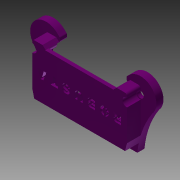
# Autodesk Inventor part: bawahbelakangbaru
Saved by Autodesk Inventor 2015 (Build 190159000, 159)
## iProperties
Created: 2015-01-14
Part Number: bawahbelakangbaru
Material: Generic
Document SubType Name: Modeling
Designer: Rafi Kurnia Putra
Density: 1 g/cm^3
Appearance: Smooth - Purple
Author: Rafi Kurnia Putra
Autodesk Inventor part; units mm, degrees
ref_plane "XY Plane" through (0, 0, 0) normal (0, 0, 1) x (1, 0, 0)
ref_plane "Work Plane2" through (0, -8.5, 0) normal (0, 1, 0) x (-1, 0, 0)
sketch "Sketch12" plane through (0, -8.5, 0) normal (0, 1, 0) x (-1, 0, 0)
  arc A0 (-42.164541, 21.859238) -> (-43.399977, 26.523474) centre (-134.113763, 0) ccw
  line L0 (0.000001, 18.359238) -> (-41.402253, 18.359238)
  arc A1 (-44.972913, 18.359238) -> (-46.899977, 26.017459) centre (-134.113763, 0) ccw
  line L1 (-43.399977, 53.851002) -> (-43.399977, 26.523474)
  line L2 (-46.899977, 36.417593) -> (-46.899977, 56.643984)
  arc A2 (-43.399977, 53.851002) -> (-40.169234, 65.136621) centre (-46.649977, 60.886625) ccw
  line L3 (-40.169234, 65.136621) -> (-34.950271, 65.136621)
  line L4 (-46.764402, 66.336532) -> (-46.764402, 65.135084)
  line L5 (-44.766541, 68.336531) -> (-36.708427, 68.345149)
  arc A3 (-44.766541, 68.336531) -> (-46.764402, 66.336532) centre (-44.764402, 66.336532) ccw
  arc A4 (-36.708427, 68.345149) -> (-33.606775, 65.655062) centre (0.000005, 107.536576) ccw
  arc A5 (-34.950271, 65.136621) -> (-33.606775, 65.655062) centre (-34.950271, 67.136621) ccw
  line L6 (0, 0) -> (0, 3.949172) construction
  line L7 (-0.000001, 18.359238) -> (41.402253, 18.359238)
  arc A6 (46.899977, 26.017459) -> (44.972913, 18.359238) centre (134.113763, 0) ccw
  line L8 (43.399977, 53.851002) -> (43.399977, 26.523474)
  line L9 (46.899977, 36.417593) -> (46.899977, 56.643984)
  arc A7 (40.169234, 65.136621) -> (43.399977, 53.851002) centre (46.649977, 60.886625) ccw
  arc A8 (46.764402, 65.135084) -> (46.899977, 56.643984) centre (46.649977, 60.886624) ccw
  line L10 (40.169234, 65.136621) -> (34.950271, 65.136621)
  line L11 (46.764402, 66.336532) -> (46.764402, 65.135084)
  line L12 (44.766541, 68.336531) -> (36.708427, 68.345149)
  arc A9 (46.764402, 66.336532) -> (44.766541, 68.336531) centre (44.764402, 66.336532) ccw
  arc A10 (33.606775, 65.655062) -> (36.708427, 68.345149) centre (-0.000005, 107.536576) ccw
  arc A11 (33.606775, 65.655062) -> (34.950271, 65.136621) centre (34.950271, 67.136621) ccw
  line L13 (-46.899977, 36.417593) -> (-46.899977, 26.017459)
  line L14 (-44.972913, 18.359238) -> (-41.402253, 18.359238)
  line L15 (41.402253, 18.359238) -> (44.972913, 18.359238)
  line L16 (0.000001, 21.859238) -> (-41.402253, 21.859238)
  line L17 (-0.000001, 21.859238) -> (41.402253, 21.859238)
  line L18 (-41.402253, 21.859238) -> (-42.164541, 21.859238)
  line L19 (41.402253, 21.859238) -> (42.164541, 21.859238)
  arc A12 (43.399977, 26.523474) -> (42.164541, 21.859238) centre (134.113763, 0) ccw
  line L20 (46.899977, 36.417593) -> (46.899977, 26.017459)
  arc A13 (-46.899977, 56.643984) -> (-46.764402, 65.135084) centre (-46.649977, 60.886624) ccw
  line L21 (-44.972913, 18.359238) -> (44.972913, 18.359238)
  line L22 (-42.164541, 21.859238) -> (42.164541, 21.859238)
  arc A14 (-44.972913, 18.359238) -> (-46.899977, 26.017459) centre (-134.113763, 0) ccw
  line L23 (-46.899977, 26.017459) -> (-46.899977, 56.643984)
  arc A15 (-46.899977, 56.643984) -> (-46.764402, 65.135084) centre (-46.649977, 60.886624) ccw
  line L24 (-46.764402, 65.135084) -> (-46.764402, 66.336532)
  arc A16 (-44.766541, 68.336531) -> (-46.764402, 66.336532) centre (-44.764402, 66.336532) ccw
  line L25 (-44.766541, 68.336531) -> (-36.708427, 68.345149)
  arc A17 (-36.708427, 68.345149) -> (-33.606775, 65.655062) centre (0.000005, 107.536576) ccw
  arc A18 (-34.950271, 65.136621) -> (-33.606775, 65.655062) centre (-34.950271, 67.136621) ccw
  line L26 (-34.950271, 65.136621) -> (-40.169234, 65.136621)
  arc A19 (-43.399977, 53.851002) -> (-40.169234, 65.136621) centre (-46.649977, 60.886625) ccw
  line L27 (-43.399977, 53.851002) -> (-43.399977, 26.523474)
  arc A20 (-42.164541, 21.859238) -> (-43.399977, 26.523474) centre (-134.113763, 0) ccw
  line L28 (-42.164541, 21.859238) -> (42.164541, 21.859238)
  arc A21 (43.399977, 26.523465) -> (42.164541, 21.859238) centre (134.110216, 0.000886) ccw
  line L29 (43.399977, 26.523465) -> (43.399977, 53.851002)
  arc A22 (40.169234, 65.136621) -> (43.399977, 53.851002) centre (46.649977, 60.886625) ccw
  line L30 (40.169234, 65.136621) -> (34.950271, 65.136621)
  arc A23 (33.606775, 65.655062) -> (34.950271, 65.136621) centre (34.950271, 67.136621) ccw
  arc A24 (33.606775, 65.655062) -> (36.708427, 68.345149) centre (-0.000005, 107.536576) ccw
  line L31 (36.708427, 68.345149) -> (44.766541, 68.336531)
  arc A25 (46.764402, 66.336532) -> (44.766541, 68.336531) centre (44.764402, 66.336532) ccw
  line L32 (46.764402, 66.336532) -> (46.764402, 65.135084)
  arc A26 (46.764402, 65.135084) -> (46.899977, 56.643984) centre (46.649977, 60.886624) ccw
  line L33 (46.899977, 56.643984) -> (46.899977, 26.017459)
  arc A27 (46.899977, 26.017459) -> (44.972913, 18.359238) centre (134.113763, 0) ccw
  line L34 (44.972913, 18.359238) -> (-44.972913, 18.359238)
  point P0 (0.000002, 53.838562)
  point P1 (-43.59264, 9.438181)
  point P2 (-46.649977, 60.886624)
  point P3 (37.970237, 69.566356)
  point P4 (-0.000002, 53.838562)
  point P5 (43.59264, 9.438181)
  point P6 (43.399975, 60.886623)
  constraints: 72 end point, 57 point on circle, 28 centre point, 22 symmetric about line, 9 tangent, 8 horizontal, 8 vertical, 4 collinear, 3 concentric, 3 parallel, 2 coincident, 1 point on line, 5 other
ref_plane "Work Plane3" through (0, -5, 0) normal (0, 1, 0) x (-1, 0, 0)
sketch "Sketch13" plane through (0, -5, 0) normal (0, 1, 0) x (-1, 0, 0)
  arc A0 (-37.970238, 69.566357) -> (-55.329713, 52.206889) centre (-46.649975, 60.886623) ccw
  arc A1 (-37.970238, 69.566357) -> (-55.329713, 52.206889) centre (-46.649975, 60.886623) ccw
  circle A2 centre (-46.649975, 60.886623) radius 3.25
  arc A3 (-40.074374, 9.438181) -> (-55.329713, 52.206889) centre (-134.113762, -0.000001) ccw
  line L0 (0.000004, 9.438181) -> (-40.074374, 9.438181)
  line L1 (0.000002, 18.359238) -> (-41.402252, 18.359238)
  arc A4 (-35.495359, 72.041226) -> (-33.611129, 70.252097) centre (0.000004, 107.536577) ccw
  arc A5 (-35.495359, 72.041226) -> (-58.067687, 50.001472) centre (-46.649975, 60.886623) ccw
  arc A6 (-43.59264, 9.438181) -> (-58.067687, 50.001472) centre (-134.113762, -0.000001) ccw
  line L2 (-43.59264, 9.438181) -> (-40.074374, 9.438181)
  line L3 (-43.399975, 53.851) -> (-43.399975, 26.523472)
  line L4 (-46.899975, 36.417593) -> (-46.899975, 56.643983)
  arc A7 (-43.399975, 53.851) -> (-40.169234, 65.136621) centre (-46.649975, 60.886623) ccw
  circle A8 centre (-46.649977, 60.886624) radius 4.25
  line L5 (-40.169234, 65.136621) -> (-34.950271, 65.136621)
  line L6 (-46.764402, 66.336532) -> (-46.764402, 65.135084)
  line L7 (-44.766541, 68.336531) -> (-36.708427, 68.345149)
  arc A9 (-44.766541, 68.336531) -> (-46.764402, 66.336532) centre (-44.764402, 66.336532) ccw
  line L8 (-32.950271, 67.136621) -> (-32.950271, 68.766601)
  arc A10 (-37.970238, 69.566357) -> (-33.606774, 65.655062) centre (0.000004, 107.536577) ccw
  arc A11 (-32.950271, 68.766601) -> (-33.611129, 70.252097) centre (-34.950271, 68.766601) ccw
  arc A12 (-34.950271, 65.136621) -> (-32.950271, 67.136621) centre (-34.950271, 67.136621) ccw
  line L9 (0, 0) -> (0, 3.949172) construction
  arc A13 (32.950271, 67.136621) -> (34.950271, 65.136621) centre (34.950271, 67.136621) ccw
  arc A14 (33.611129, 70.252097) -> (35.495359, 72.041226) centre (-0.000004, 107.536577) ccw
  line L10 (32.950271, 67.136621) -> (32.950271, 68.766601)
  arc A15 (33.611129, 70.252097) -> (32.950271, 68.766601) centre (34.950271, 68.766601) ccw
  arc A16 (33.606774, 65.655062) -> (37.970238, 69.566357) centre (-0.000004, 107.536577) ccw
  arc A17 (55.329713, 52.206889) -> (37.970238, 69.566357) centre (46.649975, 60.886623) ccw
  arc A18 (55.329713, 52.206889) -> (37.970238, 69.566357) centre (46.649975, 60.886623) ccw
  line L11 (40.169234, 65.136621) -> (34.950271, 65.136621)
  line L12 (44.766541, 68.336531) -> (36.708427, 68.345149)
  arc A19 (46.764402, 66.336532) -> (44.766541, 68.336531) centre (44.764402, 66.336532) ccw
  line L13 (46.764402, 66.336532) -> (46.764402, 65.135084)
  arc A20 (40.169234, 65.136621) -> (43.399975, 53.851) centre (46.649975, 60.886623) ccw
  circle A21 centre (46.649975, 60.886623) radius 3.25
  circle A22 centre (46.649977, 60.886624) radius 4.25
  arc A23 (58.067687, 50.001472) -> (35.495359, 72.041226) centre (46.649975, 60.886623) ccw
  arc A24 (55.329713, 52.206889) -> (40.074374, 9.438181) centre (134.113762, -0.000001) ccw
  line L14 (-0.000004, 9.438181) -> (40.074374, 9.438181)
  line L15 (-0.000002, 18.359238) -> (41.402252, 18.359238)
  line L16 (46.899975, 36.417593) -> (46.899975, 56.643983)
  line L17 (43.399975, 53.851) -> (43.399975, 26.523472)
  line L18 (43.59264, 9.438181) -> (40.074374, 9.438181)
  arc A25 (58.067687, 50.001472) -> (43.59264, 9.438181) centre (134.113762, -0.000001) ccw
  point P0 (0.000002, 53.838562)
  point P1 (-32.950271, 69.666799)
  point P2 (-43.399975, 60.886623)
  point P3 (32.950271, 69.666799)
  point P4 (43.399975, 60.886623)
  point P5 (-0.000002, 53.838562)
  constraints: 54 point on circle, 40 symmetric about line, 38 end point, 22 centre point, 12 coincident, 6 tangent, 5 vertical, 2 horizontal alignment, 2 point on line, 1 concentric, 1 horizontal, 21 other
extrude "Extrusion9" add sketch "Sketch13" along normal mid plane 7 contours A0 A3 L2 A6 A5 A4 A11 L8 A12 A10 | A24 A17 A16 A13 L10 A15 A14 A23 A25 L18
sketch "Sketch14" plane through (0, -8.5, 0) normal (0, -1, 0) x (1, 0, 0)
  line L0 (40.074374, 9.438181) -> (-40.074374, 9.438181)
  line L1 (-0.000002, 18.359238) -> (41.402252, 18.359238)
  line L2 (0.000002, 18.359238) -> (-41.402252, 18.359238)
  line L3 (-41.402252, 18.359238) -> (41.402252, 18.359238)
  arc A0 (55.329713, 52.206889) -> (40.074374, 9.438181) centre (134.113762, -0.000001) ccw
  line L4 (46.899975, 36.417593) -> (46.899975, 56.643983)
  line L5 (43.399975, 53.851) -> (43.399975, 26.523472)
  arc A1 (55.329713, 52.206889) -> (37.970238, 69.566357) centre (46.649975, 60.886623) ccw
  line L6 (44.766541, 68.336531) -> (36.708427, 68.345149)
  arc A2 (46.764402, 66.336532) -> (44.766541, 68.336531) centre (44.764402, 66.336532) ccw
  line L7 (46.764402, 66.336532) -> (46.764402, 65.135084)
  circle A3 centre (46.649975, 60.886623) radius 3.25
  arc A4 (33.606774, 65.655062) -> (37.970238, 69.566357) centre (-0.000004, 107.536577) ccw
  arc A5 (40.169234, 65.136621) -> (43.399975, 53.851) centre (46.649975, 60.886623) ccw
  line L8 (40.169234, 65.136621) -> (34.950271, 65.136621)
  arc A6 (33.606774, 65.655062) -> (34.950271, 65.136621) centre (34.950271, 67.136621) ccw
  arc A7 (55.329713, 52.206889) -> (40.074374, 9.438181) centre (134.113762, -0.000001) ccw
  arc A8 (-40.074374, 9.438181) -> (-55.329712, 52.206889) centre (-134.113762, -0.000001) ccw
  line L9 (-46.899975, 36.417593) -> (-46.899975, 56.643983)
  line L10 (-43.399975, 53.851) -> (-43.399975, 26.523472)
  arc A9 (-37.970238, 69.566357) -> (-55.329712, 52.206889) centre (-46.649975, 60.886623) ccw
  line L11 (-44.766541, 68.336531) -> (-36.708427, 68.345149)
  arc A10 (-44.766541, 68.336531) -> (-46.764401, 66.336532) centre (-44.764401, 66.336532) ccw
  line L12 (-46.764401, 66.336532) -> (-46.764401, 65.135084)
  circle A11 centre (-46.649975, 60.886623) radius 3.25
  arc A12 (-37.970238, 69.566357) -> (-33.606774, 65.655062) centre (0.000004, 107.536577) ccw
  arc A13 (-43.399975, 53.851) -> (-40.169234, 65.136621) centre (-46.649975, 60.886623) ccw
  line L13 (-40.169234, 65.136621) -> (-34.950271, 65.136621)
  arc A14 (-34.950271, 65.136621) -> (-33.606774, 65.655062) centre (-34.950271, 67.136621) ccw
  arc A15 (-40.074374, 9.438181) -> (-55.329712, 52.206889) centre (-134.113762, -0.000001) ccw
  arc A16 (46.764402, 65.135084) -> (46.899975, 56.643983) centre (46.649977, 60.886624) ccw
  arc A17 (-46.899975, 56.643983) -> (-46.764401, 65.135084) centre (-46.64998, 60.886624) ccw
  arc A18 (55.329713, 52.206889) -> (40.074374, 9.438181) centre (134.113762, -0.000001) ccw
  line L14 (40.074374, 9.438181) -> (-40.074374, 9.438181)
  arc A19 (-40.074374, 9.438181) -> (-41.402252, 18.359238) centre (-134.113732, 0.000003) ccw
  line L15 (-41.402252, 18.359238) -> (41.402252, 18.359238)
  constraints: 41 point on circle, 32 end point, 20 centre point, 4 coincident, 1 collinear, 1 horizontal
extrude "Extrusion10" add sketch "Sketch14" against normal blind 3.5 contours L0 A8 L2 L1 A0 | A0 L4 A16 L7 A2 L6 A4 A1 | A8 A9 A12 L11 A10 L12 A17 L9
extrude "Extrusion11" add sketch "Sketch12" against normal blind 13.5
sketch "Sketch16" plane through (0, -8.5, 0) normal (0, 1, 0) x (1, 0, 0)
  arc A0 (-42.164541, -21.859238) -> (-41.402252, -18.359238) centre (-134.113762, 0.000001) ccw
  line L0 (-42.164541, -21.859238) -> (42.164541, -21.859238)
  arc A1 (41.402252, -18.359238) -> (42.164541, -21.859238) centre (134.113762, 0.000001) ccw
  line L1 (41.402252, -18.359238) -> (-41.402252, -18.359238)
  arc A2 (-46.899975, -36.417593) -> (-43.399977, -26.523465) centre (-134.113762, 0.000001) ccw
  line L2 (-46.899975, -36.417593) -> (-46.899975, -56.643983)
  arc A3 (-46.764401, -65.135084) -> (-46.899975, -56.643983) centre (-46.64998, -60.886624) ccw
  line L3 (-46.764401, -65.135084) -> (-46.764401, -66.336532)
  arc A4 (-46.764401, -66.336532) -> (-44.766541, -68.336531) centre (-44.764401, -66.336532) ccw
  line L4 (-44.766541, -68.336531) -> (-36.708427, -68.345149)
  arc A5 (-33.606774, -65.655062) -> (-36.708427, -68.345149) centre (0.000004, -107.536577) ccw
  arc A6 (-33.606774, -65.655062) -> (-34.950271, -65.136621) centre (-34.950271, -67.136621) ccw
  line L5 (-34.950271, -65.136621) -> (-40.169234, -65.136621)
  arc A7 (-40.169234, -65.136621) -> (-43.399977, -53.851002) centre (-46.649977, -60.886625) ccw
  line L6 (-43.399977, -53.851002) -> (-43.399977, -26.523465)
  arc A8 (43.399977, -26.523474) -> (46.899975, -36.417593) centre (134.113762, 0.000001) ccw
  line L7 (43.399977, -26.523474) -> (43.399977, -53.851002)
  arc A9 (43.399977, -53.851002) -> (40.169234, -65.136621) centre (46.649977, -60.886625) ccw
  line L8 (40.169234, -65.136621) -> (34.950271, -65.136621)
  arc A10 (34.950271, -65.136621) -> (33.606774, -65.655062) centre (34.950271, -67.136621) ccw
  arc A11 (36.708427, -68.345149) -> (33.606774, -65.655062) centre (-0.000004, -107.536577) ccw
  line L9 (36.708427, -68.345149) -> (44.766541, -68.336531)
  arc A12 (44.766541, -68.336531) -> (46.764402, -66.336532) centre (44.764402, -66.336532) ccw
  line L10 (46.764402, -66.336532) -> (46.764402, -65.135084)
  arc A13 (46.899975, -56.643983) -> (46.764402, -65.135084) centre (46.649977, -60.886624) ccw
  line L11 (46.899975, -56.643983) -> (46.899975, -36.417593)
  point P0 (0, 0)
extrude "Extrusion12" add sketch "Sketch16" along normal blind 3.5
sketch "Sketch17" plane through (0, -22, 0) normal (0, -1, 0) x (1, 0, 0)
  line L0 (-43.399977, 26.523465) -> (-43.399977, 53.851002)
  arc A0 (-42.164541, 21.859238) -> (-43.399977, 26.523465) centre (-134.110216, 0.000886) ccw
  line L1 (42.164541, 21.859238) -> (-42.164541, 21.859238)
  arc A1 (43.399977, 26.523474) -> (42.164541, 21.859238) centre (134.113763, 0) ccw
  line L2 (43.399977, 53.851002) -> (43.399977, 26.523474)
  arc A2 (40.169234, 65.136621) -> (43.399977, 53.851002) centre (46.649977, 60.886625) ccw
  line L3 (34.950271, 65.136621) -> (40.169234, 65.136621)
  arc A3 (-43.399977, 53.851002) -> (-40.169234, 65.136621) centre (-46.649977, 60.886625) ccw
  line L4 (-40.169234, 65.136621) -> (-34.950271, 65.136621)
  line L5 (-34.950271, 65.136621) -> (34.950271, 65.136621)
  point P0 (0, 0)
  constraints: 2 end point, 1 horizontal
extrude "Extrusion13" add sketch "Sketch17" against normal blind 3.5
sketch "Sketch18" plane through (0, -22, 0) normal (0, -1, 0) x (1, 0, 0)
  line L0 (-44.972913, 18.359238) -> (44.972913, 18.359238)
  line L1 (46.899977, 26.017459) -> (46.899977, 56.643984)
  arc A0 (46.764402, 65.135084) -> (46.899977, 56.643984) centre (46.649977, 60.886624) ccw
  line L2 (46.764402, 65.135084) -> (46.764402, 66.336532)
  arc A1 (46.764402, 66.336532) -> (44.766541, 68.336531) centre (44.764402, 66.336532) ccw
  line L3 (44.766541, 68.336531) -> (36.708427, 68.345149)
  arc A2 (33.606775, 65.655062) -> (36.708427, 68.345149) centre (-0.000005, 107.536576) ccw
  arc A3 (33.606775, 65.655062) -> (34.950271, 65.136621) centre (34.950271, 67.136621) ccw
  line L4 (-34.950271, 65.136621) -> (34.950271, 65.136621)
  arc A4 (-34.950271, 65.136621) -> (-33.606775, 65.655062) centre (-34.950271, 67.136621) ccw
  arc A5 (-36.708427, 68.345149) -> (-33.606775, 65.655062) centre (0.000005, 107.536576) ccw
  line L5 (-36.708427, 68.345149) -> (-44.766541, 68.336531)
  arc A6 (-44.766541, 68.336531) -> (-46.764402, 66.336532) centre (-44.764402, 66.336532) ccw
  line L6 (-46.764402, 66.336532) -> (-46.764402, 65.135084)
  arc A7 (-46.899977, 56.643984) -> (-46.764402, 65.135084) centre (-46.649977, 60.886624) ccw
  line L7 (-46.899977, 56.643984) -> (-46.899977, 26.017459)
  arc A8 (-44.972913, 18.359238) -> (-46.899977, 26.017459) centre (-134.113763, 0) ccw
  line L8 (-44.972913, 18.359238) -> (44.972913, 18.359238)
  arc A9 (46.899977, 26.017459) -> (44.972913, 18.359238) centre (134.113763, 0) ccw
  arc A10 (46.764402, 66.336532) -> (44.766541, 68.336531) centre (44.764402, 66.336532) ccw
  line L9 (40.77767, 46.403624) -> (40.77767, 38.403624)
  line L10 (40.77767, 38.403624) -> (36.658324, 38.403624)
  spline S0 degree 2 poles (36.658324, 38.403624) (35.518767, 38.403624) (34.302212, 38.796309) (33.56304, 39.85887) (33.56304, 40.621141) knots 0 0 0 1 2 3 3 3
  spline S1 degree 2 poles (33.56304, 40.621141) (33.56304, 41.291016) (34.132819, 42.25348) (34.6256, 42.553769) knots 0 0 0 1 2 2 2
  spline S2 degree 2 poles (34.6256, 42.553769) (34.941288, 42.746261) (35.495668, 42.869457) knots 0 0 0 1 1 1
  spline S3 degree 2 poles (35.495668, 42.869457) (35.056784, 43.015751) (34.848892, 43.162046) knots 0 0 0 1 1 1
  spline S4 degree 2 poles (34.848892, 43.162046) (34.717997, 43.262142) (34.202116, 43.908918) (34.10972, 44.086011) knots 0 0 0 1 2 2 2
  line L11 (34.10972, 44.086011) -> (32.916264, 46.403624)
  line L12 (32.916264, 46.403624) -> (35.71126, 46.403624)
  line L13 (35.71126, 46.403624) -> (37.02791, 43.955116)
  spline S5 degree 2 poles (37.02791, 43.955116) (37.274301, 43.485434) (37.466794, 43.339139) knots 0 0 0 1 1 1
  spline S6 degree 2 poles (37.466794, 43.339139) (37.736284, 43.154346) (38.075071, 43.154346) knots 0 0 0 1 1 1
  line L14 (38.075071, 43.154346) -> (38.290663, 43.154346)
  line L15 (38.290663, 43.154346) -> (38.290663, 46.403624)
  line L16 (38.290663, 46.403624) -> (40.77767, 46.403624)
  line L17 (38.290663, 41.645203) -> (37.251202, 41.645203)
  spline S7 degree 2 poles (37.251202, 41.645203) (37.089508, 41.645203) (36.604426, 41.537407) knots 0 0 0 1 1 1
  spline S8 degree 2 poles (36.604426, 41.537407) (36.358035, 41.483509) (36.050047, 41.083124) (36.050047, 40.821334) knots 0 0 0 1 2 2 2
  spline S9 degree 2 poles (36.050047, 40.821334) (36.050047, 40.436348) (36.535129, 40.020564) (37.212703, 40.020564) knots 0 0 0 1 2 2 2
  line L18 (37.212703, 40.020564) -> (38.290663, 40.020564)
  line L19 (38.290663, 40.020564) -> (38.290663, 41.645203)
  spline S10 degree 2 poles (28.696822, 42.407474) (28.696822, 40.451747) (26.510104, 38.265029) (24.562077, 38.265029) knots 0 0 0 1 2 2 2
  spline S11 degree 2 poles (24.562077, 38.265029) (22.567852, 38.265029) (20.404233, 40.413249) (20.404233, 42.345876) knots 0 0 0 1 2 2 2
  spline S12 degree 2 poles (20.404233, 42.345876) (20.404233, 43.747224) (21.351298, 45.541257) (23.137631, 46.542219) (24.469681, 46.542219) knots 0 0 0 1 2 3 3 3
  spline S13 degree 2 poles (24.469681, 46.542219) (25.81713, 46.542219) (27.595764, 45.679851) (28.696822, 43.808822) (28.696822, 42.407474) knots 0 0 0 1 2 3 3 3
  spline S14 degree 2 poles (26.225215, 42.422874) (26.225215, 43.631728) (25.324349, 44.694288) (24.546678, 44.694288) knots 0 0 0 1 2 2 2
  spline S15 degree 2 poles (24.546678, 44.694288) (23.753608, 44.694288) (22.875841, 43.654827) (22.875841, 42.315078) knots 0 0 0 1 2 2 2
  spline S16 degree 2 poles (22.875841, 42.315078) (22.875841, 41.18322) (23.784407, 40.136059) (24.569777, 40.136059) knots 0 0 0 1 2 2 2
  spline S17 degree 2 poles (24.569777, 40.136059) (25.316649, 40.136059) (26.225215, 41.198619) (26.225215, 42.422874) knots 0 0 0 1 2 2 2
  line L20 (15.337823, 38.403624) -> (10.710297, 38.403624)
  spline S18 degree 2 poles (10.710297, 38.403624) (9.55534, 38.403624) (8.315686, 39.550881) (8.315686, 40.397849) knots 0 0 0 1 2 2 2
  spline S19 degree 2 poles (8.315686, 40.397849) (8.315686, 41.106223) (8.75457, 41.614404) knots 0 0 0 1 1 1
  spline S20 degree 2 poles (8.75457, 41.614404) (9.054859, 41.953191) (9.624637, 42.153384) knots 0 0 0 1 1 1
  spline S21 degree 2 poles (9.624637, 42.153384) (8.76227, 42.361276) (7.9461, 43.369938) (7.9461, 44.132209) knots 0 0 0 1 2 2 2
  spline S22 degree 2 poles (7.9461, 44.132209) (7.9461, 44.748186) (8.523579, 45.741449) (9.02406, 46.034038) knots 0 0 0 1 2 2 2
  spline S23 degree 2 poles (9.02406, 46.034038) (9.339748, 46.211132) (9.963425, 46.295828) knots 0 0 0 1 1 1
  spline S24 degree 2 poles (9.963425, 46.295828) (10.802693, 46.403624) (11.072183, 46.403624) knots 0 0 0 1 1 1
  line L21 (11.072183, 46.403624) -> (15.337823, 46.403624)
  line L22 (15.337823, 46.403624) -> (15.337823, 38.403624)
  line L23 (12.843117, 44.686589) -> (11.588064, 44.686589)
  spline S25 degree 2 poles (11.588064, 44.686589) (10.948988, 44.686589) (10.425407, 44.232306) (10.425407, 43.85502) knots 0 0 0 1 2 2 2
  spline S26 degree 2 poles (10.425407, 43.85502) (10.425407, 43.500833) (10.941288, 43.069649) (11.588064, 43.069649) knots 0 0 0 1 2 2 2
  line L24 (11.588064, 43.069649) -> (12.843117, 43.069649)
  line L25 (12.843117, 43.069649) -> (12.843117, 44.686589)
  line L26 (12.843117, 41.545106) -> (11.772857, 41.545106)
  spline S27 degree 2 poles (11.772857, 41.545106) (11.195379, 41.545106) (10.741096, 41.144721) (10.741096, 40.767436) knots 0 0 0 1 2 2 2
  spline S28 degree 2 poles (10.741096, 40.767436) (10.741096, 40.420949) (11.195379, 40.028263) (11.757457, 40.028263) knots 0 0 0 1 2 2 2
  line L27 (11.757457, 40.028263) -> (12.843117, 40.028263)
  line L28 (12.843117, 40.028263) -> (12.843117, 41.545106)
  line L29 (-2.302216, 38.403624) -> (-4.766123, 38.403624)
  line L30 (-4.766123, 38.403624) -> (-4.766123, 43.169746)
  spline S29 degree 2 poles (-4.766123, 43.169746) (-4.766123, 43.878119) (-4.32724, 45.140872) (-3.380175, 46.080236) (-2.856595, 46.272729) knots 0 0 0 1 2 3 3 3
  spline S30 degree 2 poles (-2.856595, 46.272729) (-2.140522, 46.542219) (-1.12416, 46.542219) knots 0 0 0 1 1 1
  spline S31 degree 2 poles (-1.12416, 46.542219) (-0.538982, 46.542219) (0.839267, 46.380525) (1.770932, 45.895443) (2.540903, 45.002277) (2.679498, 44.524895) knots 0 0 0 1 2 3 4 4 4
  spline S32 degree 2 poles (2.679498, 44.524895) (2.910489, 43.762623) (2.910489, 43.169746) knots 0 0 0 1 1 1
  line L31 (2.910489, 43.169746) -> (2.910489, 38.403624)
  line L32 (2.910489, 38.403624) -> (0.446581, 38.403624)
  line L33 (0.446581, 38.403624) -> (0.446581, 43.285241)
  spline S33 degree 2 poles (0.446581, 43.285241) (0.446581, 43.939717) (-0.284891, 44.678889) (-0.931667, 44.678889) knots 0 0 0 1 2 2 2
  spline S34 degree 2 poles (-0.931667, 44.678889) (-1.570743, 44.678889) (-2.302216, 43.955116) (-2.302216, 43.285241) knots 0 0 0 1 2 2 2
  line L34 (-2.302216, 43.285241) -> (-2.302216, 38.403624)
  line L35 (-9.693938, 43.754924) -> (-12.05005, 43.608629)
  spline S35 degree 2 poles (-12.05005, 43.608629) (-12.127047, 44.186107) (-12.358039, 44.486396) knots 0 0 0 1 1 1
  spline S36 degree 2 poles (-12.358039, 44.486396) (-12.743024, 44.971478) (-13.459097, 44.971478) knots 0 0 0 1 1 1
  spline S37 degree 2 poles (-13.459097, 44.971478) (-13.982678, 44.971478) (-14.560156, 44.470997) (-14.560156, 44.147609) knots 0 0 0 1 2 2 2
  spline S38 degree 2 poles (-14.560156, 44.147609) (-14.560156, 43.83962) (-14.282966, 43.59323) knots 0 0 0 1 1 1
  spline S39 degree 2 poles (-14.282966, 43.59323) (-14.013477, 43.346839) (-13.020214, 43.123547) knots 0 0 0 1 1 1
  spline S40 degree 2 poles (-13.020214, 43.123547) (-11.387875, 42.761661) (-10.694901, 42.153384) knots 0 0 0 1 1 1
  spline S41 degree 2 poles (-10.694901, 42.153384) (-9.994227, 41.545106) (-9.994227, 40.605742) knots 0 0 0 1 1 1
  spline S42 degree 2 poles (-9.994227, 40.605742) (-9.994227, 39.989765) (-10.7103, 38.896406) (-12.150146, 38.265029) (-13.3975, 38.265029) knots 0 0 0 1 2 3 3 3
  spline S43 degree 2 poles (-13.3975, 38.265029) (-14.937442, 38.265029) (-16.546682, 39.404587) (-16.700676, 40.65194) knots 0 0 0 1 2 2 2
  line L36 (-16.700676, 40.65194) -> (-14.367663, 40.790535)
  spline S44 degree 2 poles (-14.367663, 40.790535) (-14.275267, 40.251555) (-13.674689, 39.758773) (-13.151109, 39.758773) knots 0 0 0 1 2 2 2
  spline S45 degree 2 poles (-13.151109, 39.758773) (-12.719925, 39.758773) (-12.281041, 40.12066) (-12.281041, 40.39015) knots 0 0 0 1 2 2 2
  spline S46 degree 2 poles (-12.281041, 40.39015) (-12.281041, 40.574943) (-12.465835, 40.728937) knots 0 0 0 1 1 1
  spline S47 degree 2 poles (-12.465835, 40.728937) (-12.642928, 40.890631) (-13.297403, 41.021526) knots 0 0 0 1 1 1
  spline S48 degree 2 poles (-13.297403, 41.021526) (-14.922042, 41.375713) (-16.32339, 42.091786) (-16.962466, 43.146646) (-16.962466, 43.801122) knots 0 0 0 1 2 3 3 3
  spline S49 degree 2 poles (-16.962466, 43.801122) (-16.962466, 44.571093) (-16.107798, 45.872344) (-14.583255, 46.542219) (-13.412899, 46.542219) knots 0 0 0 1 2 3 3 3
  spline S50 degree 2 poles (-13.412899, 46.542219) (-11.372476, 46.542219) (-9.794035, 44.971478) (-9.693938, 43.754924) knots 0 0 0 1 2 2 2
  line L37 (-21.366701, 38.403624) -> (-28.889319, 38.403624)
  line L38 (-28.889319, 38.403624) -> (-28.889319, 40.38245)
  line L39 (-28.889319, 40.38245) -> (-26.363814, 40.38245)
  line L40 (-26.363814, 40.38245) -> (-26.363814, 46.403624)
  line L41 (-26.363814, 46.403624) -> (-23.892206, 46.403624)
  line L42 (-23.892206, 46.403624) -> (-23.892206, 40.38245)
  line L43 (-23.892206, 40.38245) -> (-21.366701, 40.38245)
  line L44 (-21.366701, 40.38245) -> (-21.366701, 38.403624)
  line L45 (-38.652553, 45.079274) -> (-35.842158, 45.079274)
  line L46 (-35.842158, 45.079274) -> (-35.449473, 46.403624)
  line L47 (-35.449473, 46.403624) -> (-32.923968, 46.403624)
  line L48 (-32.923968, 46.403624) -> (-35.934555, 38.403624)
  line L49 (-35.934555, 38.403624) -> (-38.637154, 38.403624)
  line L50 (-38.637154, 38.403624) -> (-41.640041, 46.403624)
  line L51 (-41.640041, 46.403624) -> (-39.052938, 46.403624)
  line L52 (-39.052938, 46.403624) -> (-38.652553, 45.079274)
  line L53 (-38.136672, 43.346839) -> (-37.258905, 40.474847)
  line L54 (-37.258905, 40.474847) -> (-36.381138, 43.346839)
  line L55 (-36.381138, 43.346839) -> (-38.136672, 43.346839)
  point P0 (0, 0)
  point P1 (0, 42.403624)
  point P2 (0, 42.403624)
  point P3 (0, 42.403624)
  constraints: 2 coincident, 2 other
extrude "Extrusion14" cut sketch "Sketch18" against normal through all contours L9 L10 S0 S1 S2 S3 S4 L11 L12 L13 S5 S6 L14 L15 L16 | S10 S11 S12 S13 | L20 S18 S19 S20 S21 S22 S23 S24 L21 L22 | L29 L30 S29 S30 S31 S32 L31 L32 L33 S33 S34 L34 | L35 S35 S36 S37 S38 S39 S40 S41 S42 S43 L36 S44 S45 S46 S47 S48 S49 S50 | L37 L38 L39 L40 L41 L42 L43 L44 | L45 L46 L47 L48 L49 L50 L51 L52
sketch "Sketch19" plane through (0, -22, 0) normal (0, -1, 0) x (1, 0, 0)
  line L0 (40.77767, 40.332883) -> (38.290663, 40.332883)
  line L1 (38.290663, 40.332883) -> (38.290663, 41.332883)
  line L2 (38.290663, 41.332883) -> (40.77767, 41.332883)
  line L3 (40.77767, 41.332883) -> (40.77767, 40.332883)
  line L4 (40.77767, 40.332883) -> (38.290663, 41.332883) construction
  line L5 (38.290663, 40.332883) -> (40.77767, 41.332883) construction
  spline S0 degree 2 poles (24.546678, 44.694288) (23.753608, 44.694288) (22.875841, 43.654827) (22.875841, 42.315078) knots 0 0 0 0.5 1 1 1
  spline S1 degree 2 poles (22.875841, 42.315078) (22.875841, 41.18322) (23.784407, 40.136059) (24.569777, 40.136059) knots 0 0 0 0.5 1 1 1
  spline S2 degree 2 poles (24.569777, 40.136059) (25.316649, 40.136059) (26.225215, 41.198619) (26.225215, 42.422874) knots 0 0 0 0.5 1 1 1
  spline S3 degree 2 poles (26.225215, 42.422874) (26.225215, 43.631728) (25.324349, 44.694288) (24.546678, 44.694288) knots 0 0 0 0.5 1 1 1
  spline S4 degree 2 poles (24.562077, 38.265029) (22.567852, 38.265029) (20.404233, 40.413249) (20.404233, 42.345876) knots 0 0 0 0.5 1 1 1
  spline S5 degree 2 poles (28.696822, 42.407474) (28.696822, 40.451747) (26.510104, 38.265029) (24.562077, 38.265029) knots 0 0 0 0.5 1 1 1
  line L6 (28.735321, 41.922874) -> (28.735321, 41.923109)
  line L7 (25.069777, 40.204964) -> (25.069777, 38.28474)
  line L8 (24.069777, 38.282389) -> (24.069777, 40.197708)
  line L9 (26.203703, 41.922874) -> (28.679055, 41.922874)
  line L10 (20.417845, 41.923109) -> (22.890898, 41.923109)
  line L11 (25.069777, 46.519048) -> (25.069777, 44.623804)
  line L12 (28.676972, 42.922874) -> (26.20333, 42.922874)
  line L13 (24.069777, 44.639686) -> (24.069777, 46.530347)
  line L14 (22.902236, 42.922874) -> (20.425944, 42.922874)
  spline S6 degree 2 poles (24.469681, 46.542219) (25.81713, 46.542219) (27.595764, 45.679851) (28.696822, 43.808822) (28.696822, 42.407474) knots 0 0 0 0.33333333 0.66666667 1 1 1
  spline S7 degree 2 poles (20.404233, 42.345876) (20.404233, 43.747224) (21.351298, 45.541257) (23.137631, 46.542219) (24.469681, 46.542219) knots 0 0 0 0.33333333 0.66666667 1 1 1
  line L15 (12.843117, 40.286685) -> (12.843117, 41.286685)
  line L16 (12.843117, 43.378119) -> (12.843117, 44.378119)
  line L17 (12.843117, 40.286685) -> (12.843117, 41.286685)
  line L18 (15.337823, 40.286685) -> (12.843117, 40.286685)
  line L19 (12.843117, 40.286685) -> (12.843117, 41.286685)
  line L20 (12.843117, 41.286685) -> (15.337823, 41.286685)
  line L21 (15.337823, 41.286685) -> (15.337823, 40.286685)
  line L22 (12.843117, 43.378119) -> (12.843117, 44.378119)
  line L23 (15.337823, 43.378119) -> (12.843117, 43.378119)
  line L24 (12.843117, 43.378119) -> (12.843117, 44.378119)
  line L25 (12.843117, 44.378119) -> (15.337823, 44.378119)
  line L26 (15.337823, 44.378119) -> (15.337823, 43.378119)
  line L27 (-16.700676, 40.65194) -> (-14.339333, 40.65194)
  line L28 (-16.700676, 40.65194) -> (-14.339333, 40.65194) construction
  line L29 (-16.700676, 40.65194) -> (-14.367663, 40.790535)
  line L30 (-14.339333, 40.65194) -> (-16.700676, 40.65194)
  line L31 (-16.700676, 40.65194) -> (-14.367663, 40.790535)
  line L32 (-35.842158, 45.079274) -> (-36.381138, 43.346839)
  line L33 (-36.381138, 43.346839) -> (-38.136672, 43.346839)
  line L34 (-36.381138, 43.346839) -> (-38.136672, 43.346839)
  line L35 (-38.136672, 43.346839) -> (-38.652553, 45.079274)
  line L36 (-38.652553, 45.079274) -> (-35.842158, 45.079274)
  line L37 (-35.842158, 45.079274) -> (-38.652553, 45.079274)
  arc A0 (-14.367663, 40.790535) -> (-14.339333, 40.65194) centre (-12.299592, 41.141073) ccw
  point P0 (0, 0)
  point P1 (40.77767, 40.832883)
  point P2 (39.534166, 40.832883)
  point P3 (12.843117, 38.403624)
  constraints: 70 end point, 14 parallel, 6 horizontal, 5 collinear, 2 midpoint, 2 point on circle, 1 centre point, 1 perpendicular, 1 point on line, 24 other
extrude "Extrusion15" add sketch "Sketch19" against normal blind 3.5 contours L0 L1 L2 L3 | S0 L13 S7 S6 L11 S3 | S0 S1 L10 S4 S7 L14 | L12 S6 S5 L9 S2 S3 | S1 S2 L7 S5 S4 L8 | L15 L20 L21 L18 | L16 L25 L26 L23 | L29 A0 L27 | L32 L33 L35 L36
ref_plane "Work Plane4" through (0, 0, 0) normal (1, 0, 0) x (0, 1, 0)
sketch "Sketch20" plane through (0, 0, 0) normal (1, 0, 0) x (0, 1, 0)
  line L0 (-8.5, 18.359238) -> (-22, 18.359238)
  line L1 (-8.5, 9.438181) -> (-8.5, 18.359238)
  line L2 (-8.5, 18.359238) -> (-8.5, 13.899238)
  line L3 (-8.5, 13.899238) -> (-12.96, 18.359238)
  line L4 (-12.96, 18.359238) -> (-8.5, 18.359238)
  point P0 (0, 0)
  dimension "d162" = 4.46
  dimension "d163" = 45
  constraints: 6 end point, 2 point on line, 1 perpendicular
  measures "d162" distance of L0.start L2.end
  measures "d163" angle of L2 L3
extrude "Extrusion16" add sketch "Sketch20" along normal mid plane 50
body "Solid4"
